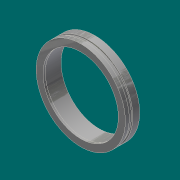
# Autodesk Inventor part: A1-19027-200-02 34in Type B victaulic ring
Saved by Autodesk Inventor 2017.3 (Build 213257000, 257)
## iProperties
Created: 2013-12-16
Part Number: A1-19027-200-02 34in Type B victaulic ring
Material: Steel, Mild
Document SubType Name: Modeling
Designer: Graeme_Van_Dongen
Density: 7.86 g/cm^3
Appearance: Steel
Description: 36" TYPE B VICTAULIC RING FOR 200 SERIES COUPLING, A350 LF2, CUSTOM TYPE B
Mass: 157165 g
Surface Area: 14200.2 cm^2
Volume: 19995.5 cm^3
Author: Graeme_Van_Dongen
Autodesk Inventor part; units mm, degrees
ref_plane "YZ Plane" through (0, 0, 0) normal (1, 0, 0) x (0, 1, 0)
ref_plane "XZ Plane" through (0, 0, 0) normal (0, 1, 0) x (-1, 0, 0)
ref_plane "XY Plane" through (0, 0, 0) normal (0, 0, 1) x (1, 0, 0)
sketch "Sketch1" plane through (0, 0, 0) normal (1, 0, 0) x (0, 1, 0)
  line L0 (412.75, 0) -> (412.75, 25.4)
  line L1 (412.75, 25.4) -> (488.95, 25.4)
  line L2 (488.95, 25.4) -> (488.95, -17.378)
  line L3 (488.95, -17.378) -> (476.25, -19.05)
  line L4 (476.25, -19.05) -> (476.25, -53.34)
  line L5 (476.25, -53.34) -> (488.95, -56.0974)
  line L6 (488.95, -56.0974) -> (488.95, -131.7625)
  line L7 (0, -218.44) -> (0, 66.04) projected
  line L8 (431.8, -144.4625) -> (431.8, -169.2731)
  line L9 (431.8, -169.2731) -> (420.6875, -177.8)
  line L10 (420.6875, -177.8) -> (419.1, -177.8)
  line L11 (419.1, -177.8) -> (419.1, -3.175)
  arc A0 (419.1, -3.175) -> (415.925, 0) centre (415.925, -3.175) ccw
  line L12 (415.925, 0) -> (412.75, 0)
  line L13 (488.95, -131.7625) -> (444.5, -131.7625)
  arc A1 (444.5, -131.7625) -> (431.8, -144.4625) centre (444.5, -144.4625) ccw
  point P0 (0, 0)
  dimension "d0" = 412.75
  dimension "d5" = 25.4
  dimension "d13" = 476.25
  dimension "d14" = 488.95
  dimension "d16" = 44.45
  dimension "d17" = 34.29
  dimension "d18" = 7.5
  dimension "d19" = 12.25
  dimension "d32" = 431.8
  dimension "d33" = 11.1125
  dimension "d35" = 1.5875
  dimension "d36" = 3.175
  dimension "d38" = 203.2
  dimension "d43" = 157.1625
  dimension "d44" = 12.7
  dimension "d45" = 90
  dimension "d46" = 37.5
  constraints: 26 end point, 4 point on circle, 4 tangent, 3 parallel, 3 perpendicular, 2 centre point, 2 vertical, 1 collinear, 1 point on line
  measures "d0" distance from line of point (0, 0) L0
  measures "d5" distance of L0.start L0.end
  measures "d13" distance from line of point (0, 0) L4
  measures "d14" distance from line of point (0, 0) L6
  measures "d16" distance from line of L3.end L1
  measures "d17" distance of L3.end L4.end
  measures "d18" angle of L1 L3
  measures "d19" angle of L5 L1
  measures "d32" distance between parallel lines of L7 L8
  measures "d33" horizontal distance of L8.end L9.end
  measures "d35" distance of L9.end L10.end
  measures "d36" radius of A0
  measures "d38" distance between parallel lines of L10 L1
  measures "d43" distance from line of L1 L6.end
  measures "d44" radius of A1
  measures "d45" angle of L6 L13
  measures "d46" angle of L9 L10
revolve "Revolution1" add sketch "Sketch1" angle 360 about axis through (0, 0, -10) along (0, 0, 1)
chamfer "Chamfer2" distance 0.7937 angle 45 1 edges at (0, -412.75, 0)
body "Solid1"
